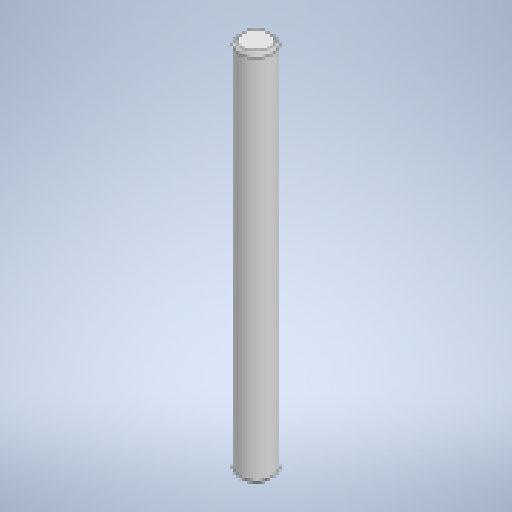
# Autodesk Inventor part: Shaft
Saved by Autodesk Inventor 2023.2 (Build 272271000, 271)
## iProperties
Created: 2023-03-04
Part Number: Shaft
Material: Generic
Document SubType Name: Modeling
Designer: Nathan Cai
Density: 1 g/cm^3
Appearance: Default
Author: Nathan Cai
Autodesk Inventor part; units mm, degrees
ref_plane "YZ Plane" through (0, 0, 0) normal (1, 0, 0) x (0, 1, 0)
ref_plane "XZ Plane" through (0, 0, 0) normal (0, 1, 0) x (-1, 0, 0)
ref_plane "XY Plane" through (0, 0, 0) normal (0, 0, 1) x (1, 0, 0)
sketch "Sketch1" plane through (0, 0, 0) normal (0, 0, 1) x (1, 0, 0)
  line L0 (0, 0) -> (2.5, 0)
  line L1 (2.5, 0) -> (2.5, 57)
  line L2 (2.5, 57) -> (0, 57)
  line L3 (0, 57) -> (0, 0)
  line L4 (2.5, 20) -> (2, 20)
  line L5 (2, 20) -> (2, 20.5)
  line L6 (2, 20.5) -> (2.5, 20.5)
  line L7 (2.5, 20.5) -> (2.5, 20)
  dimension "d0" = 2.5
  dimension "d1" = 57
  dimension "d2" = 0.5
  dimension "d3" = 0.5
  dimension "d4" = 20
  constraints: 16 end point, 4 parallel, 2 horizontal, 2 perpendicular, 1 point on line
  measures "d0" distance of L2.end L1.end
  measures "d1" distance of L1.end L0.end
  measures "d2" distance of L5.end L6.end
  measures "d3" distance of L4.end L5.end
  measures "d4" distance between parallel lines of L0 L4
revolve "Revolution1" add sketch "Sketch1" angle 360 about axis through (0, 57, 0) along (0, -1, 0) contours L3 L2 L1 L6 L5 L4 L0
chamfer "Chamfer1" distance 0.5 angle 45 2 edges at (-2.5, 57, 0) (-2.5, 0, 0)
body "Solid1"
